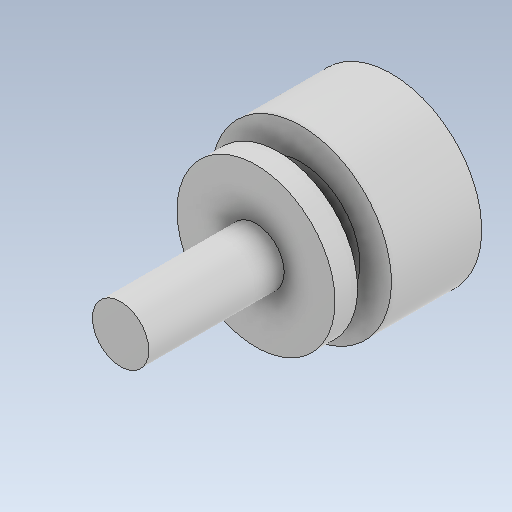
# Autodesk Inventor part: SPNFL-BRN-M3-6
Saved by Autodesk Inventor 2020.4 (Build 244396000, 396)
## iProperties
Created: 2021-09-15
Part Number: SPNFL-BRN-M3-6
Material: ステンレス鋼 AISI 304
Document SubType Name: Modeling
Designer: Masato Kubotera
Density: 8 g/cm^3
Appearance: 滑らか - 淡い灰色
Mass: 2.27476 g
Surface Area: 3.27191 cm^2
Volume: 0.284344 cm^3
Description: ネジ
Author: Masato Kubotera
Comments: https://jp.misumi-ec.com/vona2/detail/221000545997/?HissuCode=SPNFL-BRN-M3-6
Autodesk Inventor part; units mm, degrees
ref_plane "YZ Plane" through (0, 0, 0) normal (1, 0, 0) x (0, 1, 0)
ref_plane "XZ Plane" through (0, 0, 0) normal (0, 1, 0) x (-1, 0, 0)
ref_plane "XY Plane" through (0, 0, 0) normal (0, 0, 1) x (1, 0, 0)
sketch "スケッチ1" plane through (0, 0, 0) normal (0, 1, 0) x (-1, 0, 0)
  line L0 (0, 0) -> (0, 12)
  line L1 (0, 0) -> (4, 0)
  line L2 (4, 0) -> (4, 4)
  line L3 (4, 4) -> (2.6, 4)
  line L4 (2.6, 4) -> (2.6, 5) construction
  line L5 (2.6, 5) -> (3.5, 5)
  line L6 (3.5, 5) -> (3.5, 6)
  line L7 (3.5, 6) -> (1.25, 6)
  line L8 (1.25, 6) -> (1.25, 12)
  line L9 (1.25, 12) -> (0, 12)
  arc A0 (2.6, 5) -> (2.6, 4) centre (2.6, 4.5) ccw
  line L10 (2.6, 4.5) -> (2.1, 4.5) construction
  dimension "d1" = 4
  dimension "d2" = 1.25
  dimension "d3" = 3.5
  dimension "d4" = 1
  dimension "d5" = 6
  dimension "d7" = 4
  dimension "d8" = 6
  dimension "d11" = 2.1
  constraints: 22 end point, 6 perpendicular, 3 point on circle, 2 horizontal, 2 vertical, 1 centre point, 1 midpoint
  measures "d1" distance of L0.start L1.end
  measures "d2" distance of L8.end L0.end
  measures "d3" distance from line of L0.start L6
  measures "d4" distance of L5.end L6.end
  measures "d5" vertical distance of L1.end L6.end
  measures "d7" distance of L1.end L2.end
  measures "d8" distance of L7.end L8.end
  measures "d11" horizontal distance of L0.end L10.end
revolve "回転1" add sketch "スケッチ1" angle 360 about axis through (0, 0, 0) along (0, 0, 1)
